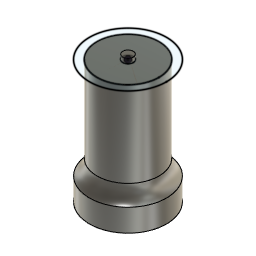
Arm Holder v2 (Autodesk Fusion 360 design; units mm, degrees)
Autodesk Fusion 360 part; units mm, degrees
sketch "Sketch1" plane through (0, 0, 0) normal (0, 0, 1) x (1, 0, 0)
  circle A0 centre (0, 0) radius 20.1
  circle A1 centre (0, 0) radius 3.4
  circle A2 centre (0, 0) radius 25
  dimension "d1" = 6.8
  dimension "d2" = 40.2
  dimension "d7" = 50
  constraint coincident A0.centre A1.centre
  constraint concentric A1 A2
  measures "d1" diameter of A1
  measures "d2" diameter of A0
  measures "d7" diameter of A2
extrude "Extrude1" add sketch "Sketch1" along normal blind 4.6 contours A2
extrude "Extrude2" add sketch "Sketch1" against normal blind 80 contours A0 | A1 | A2
extrude "Extrude3" add sketch "Sketch1" along normal blind 3 contours A1
extrude "Extrude4" cut 1 faces at (23.2736, -1.242, 4.6) along direction (0, 0, -1) blind 70
fillet "Fillet1" radius 12.5 1 edges at (-18.7398, -7.2685, -65.4)
named bodies: "Arm Holder"
